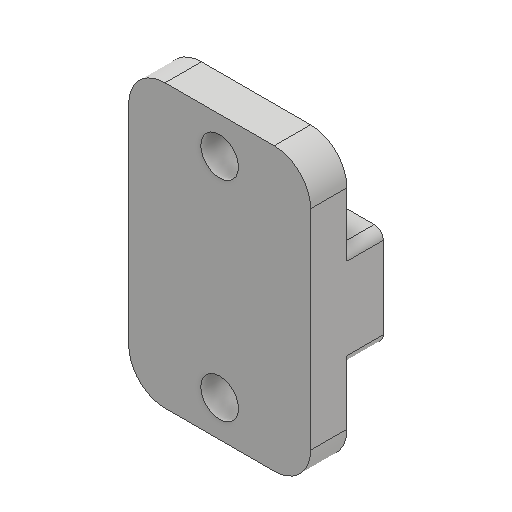
# Autodesk Inventor part: 3DP_ABS_Z_Axis_Endstop_Mount
Saved by Autodesk Inventor 2026.1 (Build 301233000, 233)
## iProperties
Created: 2015-08-14
Part Number: 3DP_ABS_Z_Axis_Endstop_Mount
Material: Ogólny
Document SubType Name: Modeling
Designer: Andrzej
Density: 1 g/cm^3
Appearance: Domyślna
Mass: 3.17828 g
Surface Area: 18.7172 cm^2
Volume: 3.17828 cm^3
Author: Andrzej
Autodesk Inventor part; units mm, degrees
ref_plane "YZ Plane" through (0, 0, 0) normal (1, 0, 0) x (0, 1, 0)
ref_plane "XZ Plane" through (0, 0, 0) normal (0, 1, 0) x (-1, 0, 0)
ref_plane "XY Plane" through (0, 0, 0) normal (0, 0, 1) x (1, 0, 0)
sketch "Szkic1" plane through (0, 0, 0) normal (0, 1, 0) x (-1, 0, 0)
  line L0 (-3.4059, 22.6049) -> (16.5941, 22.6049)
  line L1 (16.5941, 22.6049) -> (16.5941, -8.3951)
  line L2 (16.5941, -8.3951) -> (-3.4059, -8.3951)
  line L3 (-3.4059, -8.3951) -> (-3.4059, 22.6049)
  point P0 (0, 0)
  dimension "d0" = 20
  dimension "d1" = 31
  constraints: 8 end point, 2 parallel, 1 horizontal, 1 perpendicular
  measures "d0" distance of L1.end L2.end
  measures "d1" distance of L0.end L1.end
extrude "Wyciągnięcie proste1" add sketch "Szkic1" along normal blind 4
sketch "Szkic2" plane through (0, 4, 0) normal (0, 1, 0) x (1, 0, 0)
  line L0 (-16.5941, 8.3951) -> (-16.5941, -22.6049) projected
  line L1 (-16.5941, -22.6049) -> (3.4059, -22.6049) projected
  line L2 (-16.5941, -22.6049) -> (3.4059, -22.6049)
  line L3 (3.4059, -22.6049) -> (3.4059, 8.3951) projected
  line L4 (3.4059, -22.6049) -> (3.4059, 8.3951)
  line L5 (3.4059, 8.3951) -> (-16.5941, 8.3951) projected
  line L6 (3.4059, 8.3951) -> (-16.5941, 8.3951)
  line L7 (-16.5941, 8.3951) -> (-16.5941, -22.6049)
  line L8 (-16.5941, -12.6049) -> (3.4059, -12.6049)
  line L9 (-16.5941, -1.6049) -> (3.4059, -1.6049)
  point P0 (0, 0)
  point P1 (-6.5941, -18.6049)
  point P2 (-6.5941, 4.3951)
  dimension "d4" = 10
  dimension "d5" = 10
  dimension "d6" = 10
  dimension "d7" = 10
  dimension "d8" = 4
  dimension "d9" = 4
  constraints: 12 end point, 4 perpendicular, 4 point on line, 1 horizontal, 1 parallel
  measures "d4" distance between parallel lines of L5 L9
  measures "d5" distance between parallel lines of L1 L8
  measures "d6" distance from line of point (-6.594, -18.605) L0
  measures "d7" distance from line of L0 point (-6.594, 4.395)
  measures "d8" distance from line of L5 point (-6.594, 4.395)
  measures "d9" distance from line of L1 point (-6.594, -18.605)
extrude "Wyciągnięcie proste2" add sketch "Szkic2" along normal blind 4 contours L9 L3 L8 L0
fillet "Zaokrąglenie1" radius 4 4 edges at (3.4059, 2, -8.3951) (-16.5941, 2, -8.3951) (3.4059, 2, 22.6049) (-16.5941, 2, 22.6049)
hole "Otwór1" at (-6.5941, 4, 18.6049) at (-6.5941, 4, -4.3951) direction (0, -1, 0) diameter 4.15 end through all
fillet "Zaokrąglenie2" radius 1 4 edges at (3.4059, 6, 1.6049) (3.4059, 6, 12.6049) (-16.5941, 6, 1.6049) (-16.5941, 6, 12.6049)
chamfer "Faza1" distance 1 angle 45 2 edges at (-6.5941, 4, 16.5299) (-6.5941, 4, -6.4701)
